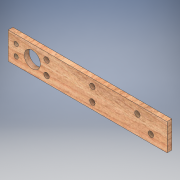
# Autodesk Inventor part: Lagerstuetze
Saved by Autodesk Inventor 2018 (Build 220112000, 112)
## iProperties
Created: 2018-01-29
Part Number: Lagerstuetze
Material: Holz (Birke)
Document SubType Name: Modeling
Designer: Julian
Density: 0.55 g/cm^3
Appearance: Birke - natur - poliert
Author: Julian
Autodesk Inventor part; units mm, degrees
ref_plane "YZ Plane" through (0, 0, 0) normal (1, 0, 0) x (0, 1, 0)
ref_plane "XZ Plane" through (0, 0, 0) normal (0, 1, 0) x (-1, 0, 0)
ref_plane "XY Plane" through (0, 0, 0) normal (0, 0, 1) x (1, 0, 0)
sketch "Skizze1" plane through (0, 0, 0) normal (0, 1, 0) x (-1, 0, 0)
  line L0 (0, 0) -> (275, 0)
  line L1 (275, 0) -> (275, -50)
  line L2 (275, -50) -> (0, -50)
  line L3 (0, -50) -> (0, 0)
  line L4 (275, 0) -> (275, -25)
  line L5 (275, -25) -> (250, -25)
  circle A0 centre (250, -25) radius 15
  line L6 (275, -50) -> (295, -50)
  line L7 (295, -50) -> (295, 0)
  line L8 (295, 0) -> (275, 0)
  dimension "d0" = 275
  dimension "d1" = 50
  dimension "d2" = 25
  dimension "d3" = 30
  dimension "d18" = 20
  constraints: 18 end point, 4 perpendicular, 2 horizontal, 2 parallel, 1 centre point, 1 coincident, 1 midpoint
  measures "d0" distance of L1.end L2.end
  measures "d1" distance of L0.end L1.end
  measures "d2" distance of L4.end L5.end
  measures "d3" diameter of A0
  measures "d18" distance of L1.end L6.end
extrude "Extrusion1" add sketch "Skizze1" along normal blind 9 contours L0 L1 L2 L3
sketch "Skizze2" plane through (0, 9, 0) normal (0, 1, 0) x (1, 0, 0)
  line L0 (0, 0) -> (0, 50) projected
  line L1 (0, 50) -> (-30, 50)
  line L2 (-30, 50) -> (-30, 35)
  line L3 (0, 0) -> (-55, 0)
  line L4 (-275, 0) -> (0, 0) projected
  line L5 (-55, 0) -> (-70, 0)
  line L6 (-70, 0) -> (-55, 0)
  line L7 (-55, 0) -> (-55, 15)
  dimension "d6" = 30
  dimension "d7" = 15
  dimension "d8" = 55
  dimension "d9" = 15
  dimension "d10" = 15
  constraints: 12 end point, 2 perpendicular, 2 point on line, 1 collinear, 1 horizontal
  measures "d6" distance of L0.end L1.end
  measures "d7" distance of L1.end L2.end
  measures "d8" distance of L0.start L3.end
  measures "d9" distance of L3.end L5.end
  measures "d10" distance of L3.end L7.end
hole "Bohrung1" at (-55, 9, -15) at (-30, 9, -35) direction (0, -1, 0) diameter 10 depth 10 tip angle 118
extrude "Extrusion2" add sketch "Skizze1" along normal blind 9 contours L8 L7 L6 L1
sketch "Skizze3" plane through (0, 0, 0) normal (0, -1, 0) x (1, 0, 0)
  line L0 (0, -50) -> (-295, -50) projected
  line L1 (-295, -50) -> (-280, -50)
  line L2 (-280, -50) -> (-280, -35)
  line L3 (-280, -35) -> (-280, -15)
  line L4 (-280, -15) -> (-280, 0)
  line L5 (-295, 0) -> (0, 0) projected
  dimension "d21" = 15
  dimension "d22" = 15
  dimension "d23" = 20
  constraints: 8 end point, 4 point on line, 1 perpendicular
  measures "d21" distance of L0.end L1.end
  measures "d22" distance of L1.end L2.end
  measures "d23" distance of L2.end L3.end
hole "Bohrung2" at (-280, 0, -15) at (-280, 0, -35) direction (0, 1, 0) diameter 8 depth 9 tip angle 118
sketch "Skizze4" plane through (0, 0, 0) normal (0, -1, 0) x (1, 0, 0)
  circle A0 centre (-250, -25) radius 15 projected
  line L0 (-250, -25) -> (-223.5, -25)
  line L1 (-223.5, -25) -> (-223.5, -37.5)
  line L2 (-223.5, -37.5) -> (-223.5, -12.5)
  line L3 (-223.5, -12.5) -> (-223.5, -25)
  line L4 (-223.5, -25) -> (-138.5, -25)
  line L5 (-138.5, -25) -> (-138.5, -37.5)
  line L6 (-138.5, -37.5) -> (-138.5, -12.5)
  point P0 (0, 0)
  dimension "d31" = 26.5
  dimension "d32" = 12.5
  dimension "d33" = 25
  dimension "d34" = 85
  dimension "d35" = 12.5
  dimension "d36" = 25
  constraints: 14 end point, 3 perpendicular, 3 point on line, 1 horizontal
  measures "d31" distance of L0.start L0.end
  measures "d32" distance of L0.end L1.end
  measures "d33" distance of L1.end L2.end
  measures "d34" distance of L0.end L4.end
  measures "d35" distance of L4.end L5.end
  measures "d36" distance of L5.end L6.end
hole "Bohrung3" at (-223.5, 0, -12.5) at (-223.5, 0, -37.5) at (-138.5, 0, -37.5) at (-138.5, 0, -12.5) direction (0, 1, 0) diameter 10 end through all
